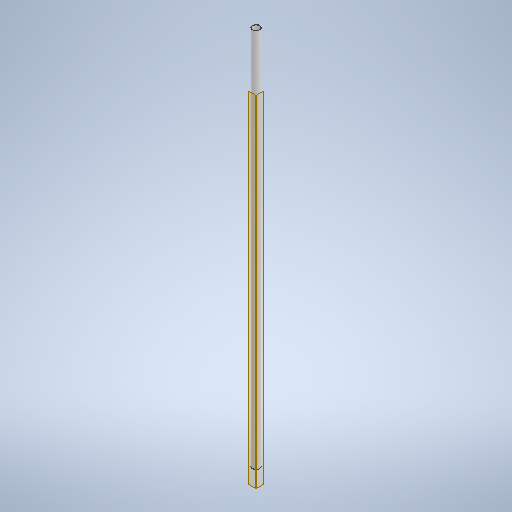
# Autodesk Inventor part: wing2
Saved by Autodesk Inventor 2025.2 (Build 292293000, 293)
## iProperties
Created: 2024-12-15
Part Number: wing2
Material: 一般
Document SubType Name: Modeling
Designer: mahhy
Density: 1 g/cm^3
Appearance: 既定
Mass: 772.95 g
Surface Area: 1156.56 cm^2
Volume: 772.95 cm^3
Author: mahhy
Autodesk Inventor part; units mm, degrees
ref_plane "XZ Plane" through (0, 0, 0) normal (0, 1, 0) x (-1, 0, 0)
sketch "スケッチ1" plane through (0, 0, 0) normal (0, 1, 0) x (-1, 0, 0)
  circle A0 centre (0, 0) radius 13.5
  dimension "d0" = 27
  constraints: 1 centre point, 1 coincident
  measures "d0" diameter of A0
extrude "押し出し1" add sketch "スケッチ1" along normal blind 1350
ref_plane "作業平面1" through (0, 0, 13.5) normal (0, 0, 1) x (1, 0, 0)
ref_plane "作業平面2" through (13.5, 0, 0) normal (1, 0, 0) x (0, 1, 0)
sketch "スケッチ2" plane through (0, 1350, 0) normal (0, 1, 0) x (1, 0, 0)
  circle A0 centre (0, 0) radius 12.5
  circle A1 centre (0, 0) radius 13.5 projected
  dimension "d5" = 25
  dimension "d6" = 1
  constraints: 1 centre point, 1 coincident
  measures "d5" diameter of A0
  measures "d6" radial gap between concentric circles of A1 A0
extrude "押し出し2" cut sketch "スケッチ2" against normal blind 1350 contours A0
